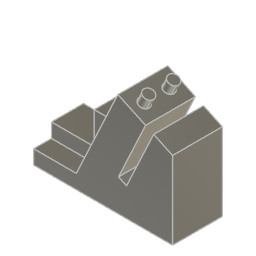
Practice problem 2 (Solid works) (Autodesk Fusion 360 design; units mm, degrees)
Autodesk Fusion 360 part; units mm, degrees
sketch "Sketch1" plane through (0, 0, 0) normal (0, 1, 0) x (1, 0, 0)
  line L0 (0, 0) -> (78, 0)
  line L1 (0, 0) -> (0, -8)
  line L2 (0, -8) -> (24, -8)
  line L3 (24, -8) -> (47.3154, -58)
  line L4 (47.3154, -58) -> (62.8659, -50.7487)
  line L5 (47.6516, -18.1216) -> (52.1832, -16.0085)
  line L6 (52.1832, -16.0085) -> (67.3974, -48.6356)
  line L7 (78, 0) -> (78, -43.6915)
  line L8 (67.3974, -48.6356) -> (78, -43.6915)
  line L9 (0, -8) -> (0, -16)
  line L10 (0, -16) -> (24, -16)
  line L11 (24, -16) -> (24, -34)
  line L12 (47.6516, -18.1216) -> (62.8659, -50.7487)
  line L13 (24, -34) -> (36.124, -34)
  dimension "d1" = 78
  dimension "d2" = 8
  dimension "d3" = 24
  dimension "d4" = 8
  dimension "d5" = 24
  dimension "d6" = 18
  dimension "d7" = 65
  dimension "d8" = 36
  dimension "d9" = 50
  dimension "d10" = 36
  dimension "d11" = 36
  dimension "d12" = 5
  dimension "d13" = 17.1581
  constraint coincident L0.start L1.start
  constraint horizontal L0
  constraint perpendicular L0 L1
  constraint perpendicular L1 L2
  constraint perpendicular L3 L4
  constraint perpendicular L4 L6
  constraint perpendicular L0 L7
  constraint perpendicular L6 L8
  constraint perpendicular L2 L9
  constraint perpendicular L9 L10
  constraint perpendicular L10 L11
  constraint perpendicular L4 L12
  constraint coincident L3 L13.end
  constraint perpendicular L11 L13
  measures "d1" distance of L0.start L0.end
  measures "d2" distance of L0.start L1.end
  measures "d3" distance of L1.end L2.end
  measures "d4" distance of L1.end L9.end
  measures "d5" distance of L9.end L10.end
  measures "d6" distance of L10.end L11.end
  measures "d7" angle of L0 L3
  measures "d8" distance of L5.end L6.end
  measures "d9" vertical distance of L2.end L3.end
  measures "d10" distance of L4.end L5.start
  measures "d11" distance of L5.start L4.end
  measures "d12" distance of L5.start L5.end
  measures "d13" distance of L3.end L4.end
extrude "Extrude1" add sketch "Sketch1" along normal blind 28
sketch "Sketch2" plane through (0, 0, 0) normal (0, -1, 0) x (1, 0, 0)
  line L0 (0, 16) -> (0, 0)
  line L1 (0, 0) -> (78, 0)
  line L2 (78, 0) -> (78, 43.6915)
  line L3 (78, 43.6915) -> (67.3974, 48.6356)
  line L4 (67.3974, 48.6356) -> (52.1832, 16.0085)
  line L5 (52.1832, 16.0085) -> (47.6516, 18.1216)
  line L6 (47.6516, 18.1216) -> (62.8659, 50.7487)
  line L7 (62.8659, 50.7487) -> (47.3154, 58)
  line L8 (47.3154, 58) -> (36.124, 34)
  line L9 (36.124, 34) -> (24, 34)
  line L10 (24, 34) -> (24, 16)
  line L11 (24, 16) -> (0, 16)
  line L12 (0, 0) -> (24, 0) construction
  line L13 (24, 0) -> (24, 8) construction
  line L14 (24, 16) -> (0, 16) construction
  line L15 (0, 16) -> (0, 0) construction
  line L16 (24, 0) -> (0, 0) construction
  line L17 (0, 0) -> (0, 8) construction
  line L18 (0, 8) -> (24, 8) construction
  line L19 (24, 8) -> (24, 0) construction
  line L20 (24, 16) -> (24, 34) construction
  line L21 (24, 34) -> (36.124, 34) construction
  line L22 (36.124, 34) -> (24, 8) construction
  line L23 (0, 8) -> (0, 16)
  line L24 (0, 16) -> (24, 16)
  line L25 (24, 16) -> (24, 34)
  line L26 (24, 34) -> (36.124, 34)
  line L27 (36.124, 34) -> (24, 8)
  line L28 (24, 8) -> (0, 8)
  dimension "d16" = 8
  constraint horizontal L12
  constraint vertical L13
  constraint horizontal L14
  constraint vertical L15
  constraint coincident L10.end L11.start
  constraint coincident L0.end L1.start
  constraint horizontal L16
  constraint vertical L17
  constraint horizontal L18
  constraint vertical L19
  constraint midpoint L15 L17.end
  constraint coincident L9.end L10.start
  constraint coincident L8.end L9.start
  constraint perpendicular L14 L23
  measures "d16" distance of L17.end L0.start
extrude "Extrude2" cut sketch "Sketch2" against normal blind 10 contours L0 L9 L10 L11 L23 L24 L25 L26 L27 L28
sketch "Sketch3" plane through (30.6661, 0, 65.7637) normal (0.422618, 0, 0.906308) x (0, 1, 0)
  line L0 (0, -18.3704) -> (0, -35.5285)
  line L1 (0, -35.5285) -> (28, -35.5285)
  line L2 (28, -35.5285) -> (28, -18.3704)
  line L3 (28, -18.3704) -> (0, -18.3704)
  line L4 (0, -18.3704) -> (28, -18.3704) construction
  line L5 (28, -18.3704) -> (28, -35.5285) construction
  line L6 (28, -35.5285) -> (0, -35.5285) construction
  line L7 (0, -35.5285) -> (0, -18.3704) construction
  line L8 (0, -35.5285) -> (28, -35.5285) construction
  line L9 (28, -35.5285) -> (28, -26.9495) construction
  line L10 (28, -26.9495) -> (0, -26.9495) construction
  line L11 (0, -26.9495) -> (0, -35.5285) construction
  line L12 (0, -26.9495) -> (28, -26.9495) construction
  line L13 (28, -26.9495) -> (28, -34.4495) construction
  line L14 (28, -34.4495) -> (0, -34.4495) construction
  line L15 (0, -34.4495) -> (0, -26.9495) construction
  line L16 (0, -26.9495) -> (28, -26.9495) construction
  line L17 (28, -26.9495) -> (28, -19.4495) construction
  line L18 (28, -19.4495) -> (0, -19.4495) construction
  line L19 (0, -19.4495) -> (0, -26.9495) construction
  line L20 (0, -35.5285) -> (7, -35.5285) construction
  line L21 (7, -35.5285) -> (7, -18.3704) construction
  line L22 (7, -18.3704) -> (0, -18.3704) construction
  line L23 (0, -18.3704) -> (0, -35.5285) construction
  line L24 (28, -35.5285) -> (21, -35.5285) construction
  line L25 (21, -35.5285) -> (21, -18.3704) construction
  line L26 (21, -18.3704) -> (28, -18.3704) construction
  line L27 (28, -18.3704) -> (28, -35.5285) construction
  circle A0 centre (7, -26.9495) radius 3
  circle A1 centre (21, -26.9495) radius 3
  dimension "d19" = 28
  dimension "d20" = 7.5
  dimension "d21" = 28
  dimension "d22" = 7.5
  dimension "d23" = 7
  dimension "d24" = 7
  dimension "d25" = 6
  dimension "d26" = 6
  constraint horizontal L4
  constraint vertical L5
  constraint horizontal L6
  constraint vertical L7
  constraint coincident L1.end L2.start
  constraint coincident L0.start L3.end
  constraint horizontal L8
  constraint vertical L9
  constraint horizontal L10
  constraint vertical L11
  constraint midpoint L5 L9.end
  constraint coincident L0.end L1.start
  constraint horizontal L12
  constraint vertical L13
  constraint horizontal L14
  constraint vertical L15
  constraint horizontal L16
  constraint vertical L17
  constraint horizontal L18
  constraint vertical L19
  constraint horizontal L20
  constraint vertical L21
  constraint horizontal L22
  constraint vertical L23
  constraint horizontal L24
  constraint vertical L25
  constraint horizontal L26
  constraint vertical L27
  constraint midpoint L21 A0.centre
  constraint midpoint L25 A1.centre
  measures "d19" distance of L10.end L9.end
  measures "d20" distance of L10.end L14.end
  measures "d21" distance of L10.end L9.end
  measures "d22" distance of L10.end L18.end
  measures "d23" distance of L0.end L20.end
  measures "d24" distance of L1.end L24.end
  measures "d25" diameter of A0
  measures "d26" diameter of A1
extrude "Extrude3" add sketch "Sketch3" along normal blind 6 contours A0 | A1
